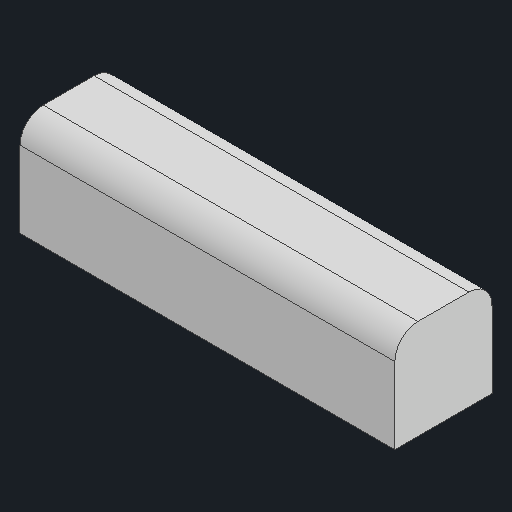
# Autodesk Inventor part: 배터리+홀더
Saved by Autodesk Inventor 2027.1 (Build 311270010, 270A)
## iProperties
Created: 2026-08-07
Part Number: 배터리+홀더
Material: 일반
Document SubType Name: Modeling
Designer: moieboy9999
Density: 1.68236 g/cm^3
Appearance: 기본값
Mass: 60 g
Surface Area: 74.7229 cm^2
Volume: 35.6643 cm^3
Author: moieboy9999
Autodesk Inventor part; units mm, degrees
ref_plane "YZ Plane" through (0, 0, 0) normal (1, 0, 0) x (0, 1, 0)
ref_plane "XZ Plane" through (0, 0, 0) normal (0, 1, 0) x (-1, 0, 0)
ref_plane "XY Plane" through (0, 0, 0) normal (0, 0, 1) x (1, 0, 0)
sketch "스케치1" plane through (0, 0, 0) normal (1, 0, 0) x (0, 1, 0)
  line L0 (0, 0) -> (21.5, 0)
  line L1 (21.5, 0) -> (21.5, -21)
  line L2 (21.5, -21) -> (0, -21)
  line L3 (0, -21) -> (0, 0)
  dimension "d0" = 21.5
  dimension "d1" = 21
  constraints: 8 end point, 2 parallel, 1 horizontal, 1 perpendicular
  measures "d0" distance of L1.end L2.end
  measures "d1" distance of L0.end L1.end
extrude "돌출1" add sketch "스케치1" along normal blind 81
fillet "모깎기1" radius 5 2 edges at (40.5, 21.5, 0) (40.5, 21.5, -21)
sketch "스케치2" plane through (0, 0, -21) normal (0, -1, 0) x (1, 0, 0)
  point P0 (0, 21)
sketch "스케치3" plane through (0, 0, -21) normal (0, -1, 0) x (1, 0, 0)
  line L0 (0, 0) -> (81, 0) projected
  line L1 (40.5, 0) -> (40.5, 10.5)
  line L2 (0, 21) -> (81, 21) projected
  circle A0 centre (40.5, 10.5) radius 1.25
  line L3 (40.5, 10.5) -> (68.5, 10.5)
  circle A1 centre (68.5, 10.5) radius 1.5
  line L4 (40.5, 10.5) -> (12.5, 10.5)
  circle A2 centre (12.5, 10.5) radius 1.5
  dimension "d5" = 10.5
  dimension "d6" = 2.5
  dimension "d7" = 28
  dimension "d8" = 3
  dimension "d9" = 28
  dimension "d10" = 3
  constraints: 6 end point, 3 centre point, 3 coincident, 2 perpendicular, 1 horizontal, 1 midpoint
  measures "d5" distance of L1.start L1.end
  measures "d6" diameter of A0
  measures "d7" distance of L3.start L3.end
  measures "d8" diameter of A1
  measures "d9" distance of L3.start L4.end
  measures "d10" diameter of A2
extrude "돌출2" cut sketch "스케치3" against normal blind 2
